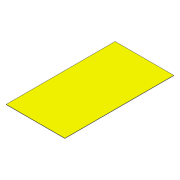
# Autodesk Inventor part: Papier Teamfarbe
Saved by Autodesk Inventor 2022.1 (Build 261234020, 234B)
## iProperties
Part Number: Papier Teamfarbe
Material: Generisch
Document SubType Name: Modeling
Designer: rYan
Density: 1 g/cm^3
Appearance: Vorgabe
Author: rYan
Autodesk Inventor part; units mm, degrees
ref_plane "YZ Plane" through (0, 0, 0) normal (1, 0, 0) x (0, 1, 0)
ref_plane "XZ Plane" through (0, 0, 0) normal (0, 1, 0) x (-1, 0, 0)
ref_plane "XY Plane" through (0, 0, 0) normal (0, 0, 1) x (1, 0, 0)
sketch "Skizze1" plane through (0, 0, 0) normal (0, 0, 1) x (1, 0, 0)
  line L0 (-28, -52) -> (28, -52)
  line L1 (28, -52) -> (28, 52)
  line L2 (28, 52) -> (-28, 52)
  line L3 (-28, 52) -> (-28, -52)
  line L4 (-28, -52) -> (28, 52) construction
  line L5 (28, -52) -> (-28, 52) construction
  point P0 (0, 0)
  dimension "d0" = 56
  dimension "d1" = 104
  constraints: 12 end point, 2 midpoint, 2 parallel, 1 horizontal, 1 perpendicular
  measures "d0" distance of L1.end L2.end
  measures "d1" distance of L0.end L1.end
extrude "Extrusion1" add sketch "Skizze1" along normal blind 0.25
